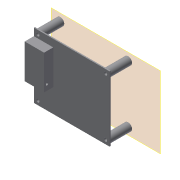
# Autodesk Inventor part: 00_Anybeam_Nebra_HAT
Saved by Autodesk Inventor 2019.4 (Build 234330000, 330)
## iProperties
Created: 2020-10-22
Part Number: 00_Anybeam_Nebra_HAT
Material: Generic
Document SubType Name: Modeling
Designer: diederichbenedict
Density: 1 g/cm^3
Appearance: Default
Author: diederichbenedict
Autodesk Inventor part; units mm, degrees
ref_plane "YZ Plane" through (0, 0, 0) normal (1, 0, 0) x (0, 1, 0)
ref_plane "XZ Plane" through (0, 0, 0) normal (0, 1, 0) x (-1, 0, 0)
ref_plane "XY Plane" through (0, 0, 0) normal (0, 0, 1) x (1, 0, 0)
ref_plane "Work Plane1" through (0, 0, 0) normal (0, 0, 1) x (1, 0, 0)
sketch "Sketch1" plane through (0, 0, 0) normal (0, 0, 1) x (1, 0, 0)
  circle A0 centre (3.51, 3.51) radius 1.375 projected
  circle A1 centre (3.51, 52.51) radius 1.375 projected
  circle A2 centre (61.51, 3.51) radius 1.375 projected
  circle A3 centre (61.51, 52.51) radius 1.375 projected
  arc A4 (81.9342, 0.01) -> (84.9342, 3.01) centre (81.9342, 3.01) ccw projected
  line L0 (84.9342, 53.01) -> (84.9342, 3.01) projected
  arc A5 (84.9342, 53.01) -> (81.9342, 56.01) centre (81.9342, 53.01) ccw projected
  line L1 (3.01, 56.01) -> (81.9342, 56.01) projected
  arc A6 (3.01, 56.01) -> (0.01, 53.01) centre (3.01, 53.01) ccw projected
  line L2 (0.01, 3.01) -> (0.01, 53.01) projected
  arc A7 (0.01, 3.01) -> (3.01, 0.01) centre (3.01, 3.01) ccw projected
  line L3 (81.9342, 0.01) -> (3.01, 0.01) projected
  circle A8 centre (62.7211, 47.7874) radius 0.5 projected
  circle A9 centre (60.1799, 47.7874) radius 0.5 projected
  circle A10 centre (17.8493, 49.9216) radius 0.2 projected
  circle A11 centre (36.5812, 39.2893) radius 0.2 projected
  circle A12 centre (37.5476, 38.3302) radius 0.2 projected
  circle A13 centre (39.0559, 38.3448) radius 0.2 projected
  circle A14 centre (40.0809, 38.3448) radius 0.2 projected
  circle A15 centre (38.7337, 39.7432) radius 0.2 projected
  circle A16 centre (39.356, 39.8091) radius 0.2 projected
  circle A17 centre (40.0296, 39.8164) radius 0.2 projected
  circle A18 centre (40.652, 39.6993) radius 0.2 projected
  circle A19 centre (41.0117, 20.1437) radius 0.2 projected
  circle A20 centre (41.1526, 21.0771) radius 0.2 projected
  circle A21 centre (40.2016, 21.3941) radius 0.2 projected
  circle A22 centre (38.7222, 22.8029) radius 0.2 projected
  circle A23 centre (41.452, 24.5993) radius 0.2 projected
  circle A24 centre (46.094, 34.1738) radius 0.2 projected
  circle A25 centre (46.11, 35.2296) radius 0.2 projected
  circle A26 centre (48.0215, 37.8609) radius 0.2 projected
  circle A27 centre (47.3576, 38.0529) radius 0.2 projected
  circle A28 centre (47.9175, 36.9172) radius 0.2 projected
  circle A29 centre (46.8138, 36.0454) radius 0.2 projected
  line L4 (46.452, 40.0993) -> (47.1053, 40.0993) projected
  line L5 (47.1053, 39.6568) -> (47.1053, 40.0993) projected
  line L6 (47.1053, 39.6568) -> (46.452, 39.6568) projected
  line L7 (46.452, 40.0993) -> (46.452, 39.6568) projected
  line L8 (46.4251, 39.252) -> (47.1215, 39.252) projected
  line L9 (47.1215, 38.669) -> (47.1215, 39.252) projected
  line L10 (47.1215, 38.669) -> (46.4251, 38.669) projected
  line L11 (46.4251, 39.252) -> (46.4251, 38.669) projected
  circle A30 centre (12.8532, 47.0439) radius 0.2 projected
  circle A31 centre (5.3847, 46.2615) radius 0.2 projected
  circle A32 centre (5.029, 47.2573) radius 0.2 projected
  circle A33 centre (7.2696, 46.5104) radius 0.2 projected
  circle A34 centre (5.1535, 44.6611) radius 0.2 projected
  circle A35 centre (5.5447, 43.203) radius 0.2 projected
  circle A36 centre (5.7581, 42.4739) radius 0.2 projected
  circle A37 centre (14.0851, 44.6759) radius 0.2 projected
  circle A38 centre (14.166, 45.5261) radius 0.2 projected
  circle A39 centre (13.0628, 44.5342) radius 0.2 projected
  circle A40 centre (37.5714, 47.3662) radius 0.2 projected
  circle A41 centre (17.0041, 47.6564) radius 0.2 projected
  circle A42 centre (16.08, 48.5805) radius 0.2 projected
  circle A43 centre (20.2948, 49.6511) radius 0.2 projected
  circle A44 centre (19.8102, 47.3409) radius 0.2 projected
  circle A45 centre (17.7479, 46.9239) radius 0.2 projected
  circle A46 centre (18.3339, 46.2027) radius 0.2 projected
  circle A47 centre (18.1649, 45.4138) radius 0.2 projected
  circle A48 centre (18.1311, 44.7489) radius 0.2 projected
  circle A49 centre (19.3482, 45.0419) radius 0.2 projected
  circle A50 centre (22.5712, 45.549) radius 0.2 projected
  circle A51 centre (22.4585, 43.2275) radius 0.2 projected
  circle A52 centre (20.2159, 42.1457) radius 0.2 projected
  circle A53 centre (21.0611, 42.1457) radius 0.2 projected
  circle A54 centre (22.9995, 39.7903) radius 0.2 projected
  circle A55 centre (24.9716, 40.7032) radius 0.2 projected
  circle A56 centre (24.1377, 41.8527) radius 0.2 projected
  circle A57 centre (26.2225, 45.0081) radius 0.2 projected
  circle A58 centre (28.7244, 47.7917) radius 0.2 projected
  circle A59 centre (29.7799, 44.7027) radius 0.2 projected
  circle A60 centre (26.4936, 42.0617) radius 0.2 projected
  circle A61 centre (27.2653, 42.0617) radius 0.2 projected
  circle A62 centre (28.1501, 41.7889) radius 0.2 projected
  circle A63 centre (28.5891, 44.6362) radius 0.2 projected
  circle A64 centre (41.8541, 33.8303) radius 0.2 projected
  circle A65 centre (39.0881, 33.1764) radius 0.2 projected
  circle A66 centre (39.2384, 32.3947) radius 0.2 projected
  circle A67 centre (37.5172, 32.7555) radius 0.2 projected
  circle A68 centre (37.5548, 31.1696) radius 0.2 projected
  circle A69 centre (37.1489, 32.2143) radius 0.2 projected
  circle A70 centre (38.9002, 30.9591) radius 0.2 projected
  circle A71 centre (47.0528, 27.6624) radius 0.2 projected
  circle A72 centre (46.4175, 27.734) radius 0.2 projected
  circle A73 centre (45.7286, 27.6892) radius 0.2 projected
  circle A74 centre (46.8112, 29.1834) radius 0.2 projected
  circle A75 centre (45.9523, 29.1834) radius 0.2 projected
  circle A76 centre (45.8002, 30.6954) radius 0.2 projected
  circle A77 centre (39.8415, 32.4043) radius 0.2 projected
  circle A78 centre (45.1292, 30.6954) radius 0.2 projected
  circle A79 centre (44.6281, 30.1407) radius 0.2 projected
  circle A80 centre (11.6818, 11.7476) radius 0.2 projected
  circle A81 centre (9.0575, 7.6392) radius 0.2 projected
  circle A82 centre (10.5992, 8.0511) radius 0.2 projected
  circle A83 centre (9.3108, 11.4405) radius 0.2 projected
  circle A84 centre (24.4942, 19.3962) radius 0.2 projected
  circle A85 centre (23.8972, 20.7096) radius 0.2 projected
  circle A86 centre (23.7266, 21.6478) radius 0.2 projected
  circle A87 centre (20.298, 18.9527) radius 0.2 projected
  circle A88 centre (19.6328, 19.9762) radius 0.2 projected
  circle A89 centre (20.2639, 22.6201) radius 0.2 projected
  circle A90 centre (21.2191, 16.0359) radius 0.2 projected
  circle A91 centre (19.7863, 17.0082) radius 0.2 projected
  circle A92 centre (16.0388, 20.435) radius 0.2 projected
  circle A93 centre (15.5322, 21.0917) radius 0.2 projected
  circle A94 centre (15.0443, 19.9472) radius 0.2 projected
  circle A95 centre (12.8303, 17.8457) radius 0.2 projected
  circle A96 centre (12.9991, 14.1306) radius 0.2 projected
  circle A97 centre (12.8115, 21.2981) radius 0.2 projected
  circle A98 centre (10.8789, 20.754) radius 0.2 projected
  circle A99 centre (9.8657, 21.0542) radius 0.2 projected
  circle A100 centre (7.4264, 20.8478) radius 0.2 projected
  circle A101 centre (15.9825, 23.3996) radius 0.2 projected
  circle A102 centre (18.2528, 25.1446) radius 0.2 projected
  circle A103 centre (18.0464, 26.3642) radius 0.2 projected
  circle A104 centre (40.4141, 32.3685) radius 0.2 projected
  circle A105 centre (39.8773, 31.1696) radius 0.2 projected
  circle A106 centre (40.4499, 31.1875) radius 0.2 projected
  circle A107 centre (41.0404, 31.1964) radius 0.2 projected
  circle A108 centre (42.5704, 29.7112) radius 0.2 projected
  circle A109 centre (41.2194, 29.7381) radius 0.2 projected
  circle A110 centre (40.2263, 29.7381) radius 0.2 projected
  circle A111 centre (40.7362, 29.2907) radius 0.2 projected
  circle A112 centre (40.1636, 29.1655) radius 0.2 projected
  circle A113 centre (43.3487, 27.7698) radius 0.2 projected
  circle A114 centre (41.9799, 27.7966) radius 0.2 projected
  circle A115 centre (40.6647, 27.6982) radius 0.2 projected
  circle A116 centre (39.9579, 27.5908) radius 0.2 projected
  circle A117 centre (39.5373, 29.3444) radius 0.2 projected
  circle A118 centre (38.92, 29.2549) radius 0.2 projected
  circle A119 centre (37.2827, 29.6218) radius 0.2 projected
  circle A120 centre (36.0749, 28.4139) radius 0.2 projected
  circle A121 centre (29.1907, 24.3381) radius 0.2 projected
  circle A122 centre (27.6996, 24.2884) radius 0.2 projected
  circle A123 centre (28.4949, 23.0706) radius 0.2 projected
  circle A124 centre (14.427, 28.8264) radius 0.2 projected
  circle A125 centre (2.9207, 47.9664) radius 0.2 projected
  circle A126 centre (7.0703, 48.4466) radius 0.2 projected
  circle A127 centre (7.5505, 49.3039) radius 0.2 projected
  circle A128 centre (15.1467, 49.7326) radius 0.2 projected
  circle A129 centre (14.0493, 49.3897) radius 0.2 projected
  circle A130 centre (14.658, 47.5806) radius 0.2 projected
  circle A131 centre (12.3002, 49.4497) radius 0.2 projected
  circle A132 centre (7.7168, 40.9892) radius 0.2 projected
  circle A133 centre (10.4087, 42.9755) radius 0.2 projected
  circle A134 centre (10.2127, 42.4005) radius 0.2 projected
  circle A135 centre (10.6701, 41.9039) radius 0.2 projected
  circle A136 centre (10.1082, 41.3159) radius 0.2 projected
  circle A137 centre (13.9239, 42.1391) radius 0.2 projected
  circle A138 centre (14.0284, 41.4073) radius 0.2 projected
  circle A139 centre (12.0552, 41.2244) radius 0.2 projected
  circle A140 centre (12.6433, 40.8454) radius 0.2 projected
  circle A141 centre (8.5139, 32.5345) radius 0.2 projected
  circle A142 centre (8.2918, 33.0964) radius 0.2 projected
  circle A143 centre (12.8001, 34.4554) radius 0.2 projected
  circle A144 centre (13.5972, 34.4162) radius 0.2 projected
  circle A145 centre (9.5201, 36.5593) radius 0.2 projected
  circle A146 centre (7.5992, 37.0167) radius 0.2 projected
  circle A147 centre (11.8723, 39.2904) radius 0.2 projected
  circle A148 centre (12.7609, 39.8262) radius 0.2 projected
  circle A149 centre (14.1591, 39.8784) radius 0.2 projected
  circle A150 centre (14.146, 38.9376) radius 0.2 projected
  circle A151 centre (13.1784, 11.4642) radius 0.2 projected
  circle A152 centre (18.3991, 11.0833) radius 0.2 projected
  circle A153 centre (19.0937, 10.792) radius 0.2 projected
  circle A154 centre (20.819, 12.8086) radius 0.2 projected
  circle A155 centre (17.7493, 13.6152) radius 0.2 projected
  circle A156 centre (16.6962, 13.5928) radius 0.2 projected
  circle A157 centre (3.9784, 11.7596) radius 0.2 projected
  circle A158 centre (4.865, 11.9936) radius 0.2 projected
  circle A159 centre (1.0352, 16.5993) radius 0.2 projected
  circle A160 centre (0.9613, 17.3874) radius 0.2 projected
  circle A161 centre (1.0967, 19.5917) radius 0.2 projected
  circle A162 centre (6.3428, 16.5008) radius 0.2 projected
  circle A163 centre (6.3551, 17.8923) radius 0.2 projected
  circle A164 centre (7.1076, 30.2668) radius 0.2 projected
  circle A165 centre (7.0255, 27.339) radius 0.2 projected
  circle A166 centre (7.0392, 24.3017) radius 0.2 projected
  circle A167 centre (10.8426, 27.3527) radius 0.2 projected
  circle A168 centre (7.2488, 32.9091) radius 0.2 projected
  circle A169 centre (9.1368, 34.4688) radius 0.2 projected
  circle A170 centre (14.1852, 37.9575) radius 0.2 projected
  circle A171 centre (14.0758, 37.0956) radius 0.2 projected
  circle A172 centre (14.1579, 36.4799) radius 0.2 projected
  circle A173 centre (18.4675, 36.261) radius 0.2 projected
  circle A174 centre (19.2676, 35.2967) radius 0.2 projected
  circle A175 centre (13.3428, 33.2614) radius 0.2 projected
  circle A176 centre (13.4898, 32.4473) radius 0.2 projected
  circle A177 centre (12.6898, 32.1644) radius 0.2 projected
  circle A178 centre (11.4913, 31.1129) radius 0.2 projected
  circle A179 centre (16.4974, 28.75) radius 0.2 projected
  circle A180 centre (11.6806, 26.3755) radius 0.2 projected
  circle A181 centre (11.8276, 27.3253) radius 0.2 projected
  circle A182 centre (13.8092, 30.8641) radius 0.2 projected
  circle A183 centre (13.7407, 30.1903) radius 0.2 projected
  circle A184 centre (13.6493, 28.7855) radius 0.2 projected
  circle A185 centre (13.7635, 26.5013) radius 0.2 projected
  circle A186 centre (13.7064, 27.3236) radius 0.2 projected
  circle A187 centre (18.0693, 28.8654) radius 0.2 projected
  circle A188 centre (18.2749, 27.1865) radius 0.2 projected
  circle A189 centre (18.4233, 25.7475) radius 0.2 projected
  circle A190 centre (42.354, 45.4661) radius 0.2 projected
  circle A191 centre (43.2414, 45.549) radius 0.2 projected
  circle A192 centre (44.1537, 45.5573) radius 0.2 projected
  circle A193 centre (40.3139, 42.522) radius 0.2 projected
  circle A194 centre (42.8516, 41.6098) radius 0.2 projected
  circle A195 centre (39.4431, 43.6167) radius 0.2 projected
  circle A196 centre (40.3968, 43.5835) radius 0.2 projected
  circle A197 centre (41.5081, 43.6001) radius 0.2 projected
  circle A198 centre (84.1123, 38.0141) radius 0.2 projected
  circle A199 centre (79.6259, 38.2091) radius 0.2 projected
  circle A200 centre (48.1699, 12.8899) radius 0.2 projected
  circle A201 centre (65.0598, 17.0332) radius 0.2 projected
  circle A202 centre (64.2609, 17.846) radius 0.2 projected
  circle A203 centre (68.3812, 24.4748) radius 0.2 projected
  circle A204 centre (68.2971, 22.3026) radius 0.2 projected
  circle A205 centre (67.4983, 20.5227) radius 0.2 projected
  circle A206 centre (64.4571, 24.9933) radius 0.2 projected
  circle A207 centre (63.364, 22.1204) radius 0.2 projected
  circle A208 centre (53.5119, 27.0534) radius 0.2 projected
  circle A209 centre (55.3618, 26.0164) radius 0.2 projected
  circle A210 centre (56.1186, 28.6511) radius 0.2 projected
  circle A211 centre (57.0435, 28.609) radius 0.2 projected
  circle A212 centre (58.5431, 28.4549) radius 0.2 projected
  circle A213 centre (60.0706, 28.525) radius 0.2 projected
  circle A214 centre (60.7777, 25.9208) radius 0.2 projected
  circle A215 centre (61.0198, 26.5324) radius 0.2 projected
  circle A216 centre (62.0645, 25.8953) radius 0.2 projected
  circle A217 centre (61.7333, 26.4559) radius 0.2 projected
  circle A218 centre (61.7842, 28.5199) radius 0.2 projected
  circle A219 centre (62.6123, 28.5199) radius 0.2 projected
  circle A220 centre (63.6443, 28.609) radius 0.2 projected
  circle A221 centre (64.4229, 28.4392) radius 0.2 projected
  circle A222 centre (65.1448, 32.1056) radius 0.2 projected
  circle A223 centre (65.1732, 34.6395) radius 0.2 projected
  circle A224 centre (65.4563, 35.2765) radius 0.2 projected
  circle A225 centre (65.1448, 37.2159) radius 0.2 projected
  circle A226 centre (64.9891, 38.1502) radius 0.2 projected
  circle A227 centre (63.6585, 39.2402) radius 0.2 projected
  circle A228 centre (62.5543, 40.4151) radius 0.2 projected
  circle A229 centre (60.2327, 40.3868) radius 0.2 projected
  circle A230 centre (55.0516, 40.2452) radius 0.2 projected
  circle A231 centre (49.2898, 45.5976) radius 0.2 projected
  circle A232 centre (47.7592, 43.8525) radius 0.2 projected
  circle A233 centre (45.1074, 43.3845) radius 0.2 projected
  circle A234 centre (47.6032, 41.8636) radius 0.2 projected
  circle A235 centre (47.8469, 41.1909) radius 0.2 projected
  circle A236 centre (46.5503, 40.7327) radius 0.2 projected
  circle A237 centre (45.9653, 40.1088) radius 0.2 projected
  circle A238 centre (44.2982, 39.7578) radius 0.2 projected
  circle A239 centre (43.6547, 39.709) radius 0.2 projected
  circle A240 centre (45.162, 36.0312) radius 0.2 projected
  circle A241 centre (43.4561, 36.6901) radius 0.2 projected
  circle A242 centre (42.702, 36.0385) radius 0.2 projected
  circle A243 centre (37.7966, 35.2917) radius 0.2 projected
  circle A244 centre (40.0589, 34.684) radius 0.2 projected
  circle A245 centre (39.195, 35.1892) radius 0.2 projected
  circle A246 centre (40.1102, 35.2551) radius 0.2 projected
  circle A247 centre (38.8875, 36.2069) radius 0.2 projected
  circle A248 centre (39.4952, 36.3899) radius 0.2 projected
  circle A249 centre (40.4762, 36.324) radius 0.2 projected
  circle A250 centre (40.1687, 36.8658) radius 0.2 projected
  circle A251 centre (40.8863, 36.9683) radius 0.2 projected
  circle A252 centre (42.5702, 37.986) radius 0.2 projected
  circle A253 centre (40.3225, 37.4589) radius 0.2 projected
  circle A254 centre (37.5989, 36.756) radius 0.2 projected
  circle A255 centre (42.5556, 37.166) radius 0.2 projected
  circle A256 centre (39.0485, 37.5101) radius 0.2 projected
  circle A257 centre (11.5458, 48.2837) radius 0.2 projected
  circle A258 centre (11.6829, 47.1262) radius 0.2 projected
  circle A259 centre (12.1519, 45.2427) radius 0.2 projected
  circle A260 centre (12.1872, 44.2312) radius 0.2 projected
  circle A261 centre (11.2111, 44.243) radius 0.2 projected
  circle A262 centre (8.365, 45.4544) radius 0.2 projected
  circle A263 centre (8.4002, 44.8663) radius 0.2 projected
  circle A264 centre (8.2238, 43.8431) radius 0.2 projected
  circle A265 centre (5.9893, 41.6203) radius 0.2 projected
  circle A266 centre (11.9376, 38.0098) radius 0.2 projected
  circle A267 centre (11.6632, 36.4155) radius 0.2 projected
  circle A268 centre (6.789, 41.8908) radius 0.2 projected
  circle A269 centre (7.4947, 41.9039) radius 0.2 projected
  circle A270 centre (6.5277, 40.179) radius 0.2 projected
  circle A271 centre (6.5669, 39.3688) radius 0.2 projected
  circle A272 centre (7.0373, 38.5586) radius 0.2 projected
  circle A273 centre (7.7037, 39.3035) radius 0.2 projected
  circle A274 centre (8.723, 40.4926) radius 0.2 projected
  circle A275 centre (8.344, 39.5779) radius 0.2 projected
  circle A276 centre (7.8736, 40.2182) radius 0.2 projected
  circle A277 centre (29.1549, 13.7915) radius 0.2 projected
  circle A278 centre (27.3819, 14.6837) radius 0.2 projected
  circle A279 centre (29.0062, 15.6674) radius 0.2 projected
  circle A280 centre (29.0977, 14.5922) radius 0.2 projected
  circle A281 centre (29.052, 12.8993) radius 0.2 projected
  circle A282 centre (26.1923, 13.883) radius 0.2 projected
  circle A283 centre (25.5517, 17.4176) radius 0.2 projected
  circle A284 centre (19.1306, 7.859) radius 0.2 projected
  circle A285 centre (22.4633, 13.0937) radius 0.2 projected
  circle A286 centre (22.052, 4.6993) radius 0.2 projected
  circle A287 centre (23.0683, 2.2713) radius 0.2 projected
  circle A288 centre (22.9648, 1.2738) radius 0.2 projected
  circle A289 centre (20.7156, 1.2832) radius 0.2 projected
  circle A290 centre (18.9182, 1.2173) radius 0.2 projected
  circle A291 centre (20.5745, 4.8781) radius 0.2 projected
  circle A292 centre (17.0737, 4.0311) radius 0.2 projected
  circle A293 centre (20.1698, 6.2332) radius 0.2 projected
  circle A294 centre (16.2361, 4.1911) radius 0.2 projected
  circle A295 centre (9.7989, 7.2391) radius 0.2 projected
  circle A296 centre (3.51, 52.51) radius 1.375 projected
  circle A297 centre (3.51, 3.51) radius 1.375 projected
  circle A298 centre (61.51, 3.51) radius 1.375 projected
  circle A299 centre (61.51, 52.51) radius 1.375 projected
  circle A300 centre (9.2652, 49.8784) radius 0.2 projected
  circle A301 centre (3.51, 52.51) radius 3.375
  circle A302 centre (3.51, 3.51) radius 3.375
  circle A303 centre (61.51, 52.51) radius 3.375
  circle A304 centre (61.51, 3.51) radius 3.375
  point P0 (0, 0)
  dimension "d0" = 2
  dimension "d1" = 2
  dimension "d2" = 2
  dimension "d3" = 2
  constraints: 4 centre point
  measures "d0" radial gap between concentric circles of A1 A301
  measures "d1" radial gap between concentric circles of A0 A302
  measures "d2" radial gap between concentric circles of A3 A303
  measures "d3" radial gap between concentric circles of A2 A304
extrude "Extrusion1" add sketch "Sketch1" along normal blind 18.27 contours A301 | A302 | A303 | A304
sketch "Sketch2" plane through (3.51, 52.51, 18.27) normal (0, 0, 1) x (1, 0, 0)
  circle A0 centre (0, 0) radius 1.375 projected
  circle A1 centre (0, 0) radius 3.375 projected
  circle A2 centre (0, -49) radius 1.375 projected
  circle A3 centre (0, -49) radius 3.375 projected
  circle A4 centre (58, -49) radius 1.375 projected
  circle A5 centre (58, -49) radius 1.375 projected
  circle A6 centre (58, -49) radius 3.375 projected
  circle A7 centre (58, 0) radius 1.375 projected
  circle A8 centre (58, 0) radius 3.375 projected
  line L0 (-3.375, 0) -> (-3.375, -49)
  line L1 (0, 3.375) -> (58, 3.375)
  circle A9 centre (58, 0) radius 3.375 projected
  line L2 (61.375, 0) -> (61.375, -49)
  line L3 (58, -52.375) -> (0, -52.375)
  line L4 (-3.375, 3.375) -> (61.375, 3.375)
  line L5 (61.375, 3.375) -> (61.375, -52.375)
  line L6 (61.375, -52.375) -> (-3.375, -52.375)
  line L7 (-3.375, -52.375) -> (-3.375, 3.375)
  point P0 (-3.51, -52.51)
  constraints: 16 end point, 5 point on circle, 2 horizontal, 2 parallel, 2 perpendicular, 2 tangent, 2 vertical, 1 horizontal alignment, 1 vertical alignment, 2 other
extrude "Extrusion2" add sketch "Sketch2" along normal blind 1
sketch "Sketch3" plane through (0.135, 3.51, 18.27) normal (-1, 0, 0) x (0, 0, 1)
  line L0 (1, 52.375) -> (1, -3.375) projected
  line L1 (0, -3.375) -> (0, 0) projected
  line L2 (0, -3.375) -> (1, -3.375) projected
  line L3 (1, 52.375) -> (1, -3.375) projected
  line L4 (0, 52.375) -> (1, 52.375) projected
  line L5 (0, 49) -> (0, 52.375) projected
  line L6 (0, 0) -> (0, 49) projected
  line L7 (1, 46.075) -> (8.85, 46.075)
  line L8 (8.85, 46.075) -> (8.85, 16.625)
  line L9 (8.85, 16.625) -> (1, 16.625)
  line L10 (1, 16.625) -> (1, 46.075)
  line L11 (-19.6, 49.5) -> (-19.6, -0.5) projected
  circle A0 centre (6.3, 21.5) radius 1
  line L12 (-19.6, 52.5) -> (-18.27, 52.5) projected
  point P0 (-18.27, -3.51)
  dimension "d8" = 6.3
  dimension "d9" = 20
  dimension "d10" = 28.45
  dimension "d11" = 2
  dimension "d12" = 25.9
  dimension "d13" = 31
  constraints: 8 end point, 2 parallel, 1 centre point, 1 horizontal, 1 perpendicular, 1 point on line
  measures "d8" distance between parallel lines of L7 L4
  measures "d9" distance between parallel lines of L2 L9
  measures "d10" distance between parallel lines of L11 L8
  measures "d11" diameter of A0
  measures "d12" distance from line of A0.centre L11
  measures "d13" distance from line of A0.centre L12
extrude "Extrusion3" add sketch "Sketch3" against normal blind 16.6 contours L7 L8 L9 L0
body "Solid1"
